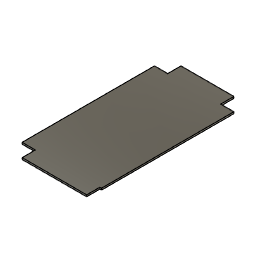
_ShelfI.5fef8cea-7e15-4213-bb0c-d7298d23d59a (Autodesk Fusion 360 design; units mm, degrees)
Autodesk Fusion 360 part; units mm, degrees
note: some values were not read from the file. Set by a fixed rule: which sketch regions a step uses.
sketch "Sketch1" plane through (0, 0, 0) normal (0, 0, 1) x (1, 0, 0)
  line L0 (0, 0) -> (0, 609.6)
  line L1 (0, 609.6) -> (304.8, 609.6)
  line L2 (304.8, 609.6) -> (304.8, 0)
  line L3 (304.8, 0) -> (0, 0)
  line L4 (0, 0) -> (50.8, 0)
  line L5 (50.8, 0) -> (50.8, 50.8)
  line L6 (50.8, 50.8) -> (0, 50.8)
  line L7 (0, 50.8) -> (0, 0)
  line L8 (0, 609.6) -> (50.8, 609.6)
  line L9 (50.8, 609.6) -> (50.8, 558.8)
  line L10 (50.8, 558.8) -> (0, 558.8)
  line L11 (0, 558.8) -> (0, 609.6)
  line L12 (304.8, 609.6) -> (254, 609.6)
  line L13 (254, 609.6) -> (254, 558.8)
  line L14 (254, 558.8) -> (304.8, 558.8)
  line L15 (304.8, 558.8) -> (304.8, 609.6)
  line L16 (304.8, 0) -> (298.45, 0)
  line L17 (298.45, 0) -> (298.45, 50.8)
  line L18 (298.45, 50.8) -> (304.8, 50.8)
  line L19 (304.8, 50.8) -> (304.8, 0)
  dimension "d2" = 609.6
  dimension "d3" = 304.8
  dimension "d10" = 50.8
  dimension "d11" = 50.8
  dimension "d12" = 50.8
  dimension "d13" = 50.8
  dimension "d14" = 6.35
  dimension "d16" = 304.8
  constraint coincident L0.start L3.end
  constraint vertical L0
  constraint perpendicular L0 L1
  constraint perpendicular L1 L2
  constraint perpendicular L0 L3
  constraint horizontal L4
  constraint vertical L5
  constraint horizontal L6
  constraint vertical L7
  constraint horizontal L8
  constraint vertical L9
  constraint horizontal L10
  constraint vertical L11
  constraint horizontal L12
  constraint vertical L13
  constraint horizontal L14
  constraint vertical L15
  constraint collinear L10 L14
  constraint collinear L5 L9
  constraint horizontal L16
  constraint vertical L17
  constraint horizontal L18
  constraint vertical L19
  constraint collinear L6 L18
  measures "d2" distance of L0.start L0.end
  measures "d3" distance of L0.end L1.end
  measures "d10" distance of L0.start L4.end
  measures "d11" distance of L1.end L14.end
  measures "d12" distance of L1.end L12.end
  measures "d13" distance of L4.end L5.end
  measures "d14" distance of L17.end L18.end
extrude "Extrude1" add sketch "Sketch1" along normal blind 6.35 contours L0 L1 L2 L3 L5 L6 L9 L10 L13 L14 L17 L18
